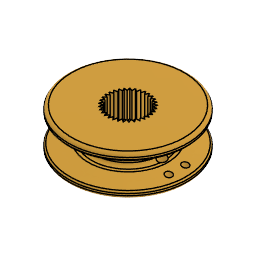
Spool_v3 (Autodesk Fusion 360 design; units mm, degrees)
Autodesk Fusion 360 part; units mm, degrees
sketch "Sketch1" plane through (0, 0, 0) normal (0, 0, 1) x (1, 0, 0)
  line L0 (-0.0246, -2.4999) -> (0.1607, -2.8207)
  line L1 (0.1607, -2.8207) -> (0.3083, -2.4809)
  arc A0 (0.3083, -2.4809) -> (0.449, -2.4594) centre (0, 0) ccw
  line L2 (0.449, -2.4594) -> (0.6916, -2.7393)
  line L3 (0.6916, -2.7393) -> (0.7722, -2.3777)
  arc A1 (0.7722, -2.3777) -> (0.9063, -2.3299) centre (0, 0) ccw
  line L4 (0.9063, -2.3299) -> (1.1975, -2.5589)
  line L5 (1.1975, -2.5589) -> (1.2083, -2.1886)
  arc A2 (1.2083, -2.1886) -> (1.3309, -2.1163) centre (0, 0) ccw
  line L6 (1.3309, -2.1163) -> (1.6601, -2.286)
  line L7 (1.6601, -2.286) -> (1.6006, -1.9204)
  arc A3 (1.6006, -1.9204) -> (1.7073, -1.8262) centre (0, 0) ccw
  line L8 (1.7073, -1.8262) -> (2.0628, -1.9306)
  line L9 (2.0628, -1.9306) -> (1.9351, -1.5828)
  arc A4 (1.9351, -1.5828) -> (2.0221, -1.4701) centre (0, 0) ccw
  line L10 (2.0221, -1.4701) -> (2.3909, -1.5053)
  line L11 (2.3909, -1.5053) -> (2.1997, -1.188)
  arc A5 (2.1997, -1.188) -> (2.2638, -1.0608) centre (0, 0) ccw
  line L12 (2.2638, -1.0608) -> (2.6325, -1.0256)
  line L13 (2.6325, -1.0256) -> (2.3848, -0.7502)
  arc A6 (2.3848, -0.7502) -> (2.4236, -0.6133) centre (0, 0) ccw
  line L14 (2.4236, -0.6133) -> (2.7791, -0.5089)
  line L15 (2.7791, -0.5089) -> (2.4837, -0.2853)
  arc A7 (2.4837, -0.2853) -> (2.4959, -0.1435) centre (0, 0) ccw
  line L16 (2.4959, -0.1435) -> (2.8251, 0.0263)
  line L17 (2.8251, 0.0263) -> (2.4928, 0.1899)
  arc A8 (2.4928, 0.1899) -> (2.4779, 0.3314) centre (0, 0) ccw
  line L18 (2.4779, 0.3314) -> (2.7691, 0.5605)
  line L19 (2.7691, 0.5605) -> (2.4118, 0.6582)
  arc A9 (2.4118, 0.6582) -> (2.3704, 0.7944) centre (0, 0) ccw
  line L20 (2.3704, 0.7944) -> (2.613, 1.0744)
  line L21 (2.613, 1.0744) -> (2.2436, 1.1028)
  arc A10 (2.2436, 1.1028) -> (2.1772, 1.2287) centre (0, 0) ccw
  line L22 (2.1772, 1.2287) -> (2.3625, 1.5495)
  line L23 (2.3625, 1.5495) -> (1.9944, 1.5074)
  arc A11 (1.9944, 1.5074) -> (1.9054, 1.6185) centre (0, 0) ccw
  line L24 (1.9054, 1.6185) -> (2.0265, 1.9686)
  line L25 (2.0265, 1.9686) -> (1.6731, 1.8576)
  arc A12 (1.6731, 1.8576) -> (1.5646, 1.9498) centre (0, 0) ccw
  line L26 (1.5646, 1.9498) -> (1.6173, 2.3165)
  line L27 (1.6173, 2.3165) -> (1.2913, 2.1407)
  arc A13 (1.2913, 2.1407) -> (1.1674, 2.2107) centre (0, 0) ccw
  line L28 (1.1674, 2.2107) -> (1.1497, 2.5807)
  line L29 (1.1497, 2.5807) -> (0.8628, 2.3464)
  arc A14 (0.8628, 2.3464) -> (0.7279, 2.3917) centre (0, 0) ccw
  line L30 (0.7279, 2.3917) -> (0.6405, 2.7517)
  line L31 (0.6405, 2.7517) -> (0.4032, 2.4673)
  arc A15 (0.4032, 2.4673) -> (0.2621, 2.4862) centre (0, 0) ccw
  line L32 (0.2621, 2.4862) -> (0.1082, 2.8232)
  line L33 (0.1082, 2.8232) -> (-0.0711, 2.499)
  arc A16 (-0.0711, 2.499) -> (-0.2132, 2.4909) centre (0, 0) ccw
  line L34 (-0.2132, 2.4909) -> (-0.4281, 2.7926)
  line L35 (-0.4281, 2.7926) -> (-0.5427, 2.4404)
  arc A17 (-0.5427, 2.4404) -> (-0.6807, 2.4055) centre (0, 0) ccw
  line L36 (-0.6807, 2.4055) -> (-0.9488, 2.6612)
  line L37 (-0.9488, 2.6612) -> (-0.9948, 2.2936)
  arc A18 (-0.9948, 2.2936) -> (-1.1237, 2.2332) centre (0, 0) ccw
  line L38 (-1.1237, 2.2332) -> (-1.4353, 2.4335)
  line L39 (-1.4353, 2.4335) -> (-1.4108, 2.0639)
  arc A19 (-1.4108, 2.0639) -> (-1.526, 1.9802) centre (0, 0) ccw
  line L40 (-1.526, 1.9802) -> (-1.8699, 2.1179)
  line L41 (-1.8699, 2.1179) -> (-1.7759, 1.7596)
  arc A20 (-1.7759, 1.7596) -> (-1.8732, 1.6556) centre (0, 0) ccw
  line L42 (-1.8732, 1.6556) -> (-2.2369, 1.7257)
  line L43 (-2.2369, 1.7257) -> (-2.0768, 1.3917)
  arc A21 (-2.0768, 1.3917) -> (-2.1527, 1.2712) centre (0, 0) ccw
  line L44 (-2.1527, 1.2712) -> (-2.5231, 1.2712)
  line L45 (-2.5231, 1.2712) -> (-2.3027, 0.9735)
  arc A22 (-2.3027, 0.9735) -> (-2.3543, 0.8409) centre (0, 0) ccw
  line L46 (-2.3543, 0.8409) -> (-2.7181, 0.7707)
  line L47 (-2.7181, 0.7707) -> (-2.4453, 0.5201)
  arc A23 (-2.4453, 0.5201) -> (-2.4709, 0.3801) centre (0, 0) ccw
  line L48 (-2.4709, 0.3801) -> (-2.8148, 0.2424)
  line L49 (-2.8148, 0.2424) -> (-2.4995, 0.0479)
  arc A24 (-2.4995, 0.0479) -> (-2.4982, -0.0944) centre (0, 0) ccw
  line L50 (-2.4982, -0.0944) -> (-2.8098, -0.2947)
  line L51 (-2.8098, -0.2947) -> (-2.4634, -0.426)
  arc A25 (-2.4634, -0.426) -> (-2.4352, -0.5655) centre (0, 0) ccw
  line L52 (-2.4352, -0.5655) -> (-2.7033, -0.8211)
  line L53 (-2.7033, -0.8211) -> (-2.3383, -0.8845)
  arc A26 (-2.3383, -0.8845) -> (-2.2842, -1.0161) centre (0, 0) ccw
  line L54 (-2.2842, -1.0161) -> (-2.499, -1.3179)
  line L55 (-2.499, -1.3179) -> (-2.1287, -1.311)
  arc A27 (-2.1287, -1.311) -> (-2.0506, -1.4301) centre (0, 0) ccw
  line L56 (-2.0506, -1.4301) -> (-2.2045, -1.767)
  line L57 (-2.2045, -1.767) -> (-1.8421, -1.6902)
  arc A28 (-1.8421, -1.6902) -> (-1.7429, -1.7923) centre (0, 0) ccw
  line L58 (-1.7429, -1.7923) -> (-1.8302, -2.1523)
  line L59 (-1.8302, -2.1523) -> (-1.4889, -2.0083)
  arc A29 (-1.4889, -2.0083) -> (-1.3722, -2.0897) centre (0, 0) ccw
  line L60 (-1.3722, -2.0897) -> (-1.3898, -2.4598)
  line L61 (-1.3898, -2.4598) -> (-1.0819, -2.2538)
  arc A30 (-1.0819, -2.2538) -> (-0.9519, -2.3117) centre (0, 0) ccw
  line L62 (-0.9519, -2.3117) -> (-0.8992, -2.6783)
  line L63 (-0.8992, -2.6783) -> (-0.6359, -2.4178)
  arc A31 (-0.6359, -2.4178) -> (-0.4972, -2.4501) centre (0, 0) ccw
  line L64 (-0.4972, -2.4501) -> (-0.3761, -2.8001)
  line L65 (-0.3761, -2.8001) -> (-0.1668, -2.4944)
  arc A32 (-0.1668, -2.4944) -> (-0.0246, -2.4999) centre (0, 0) ccw
  circle A33 centre (0, 0) radius 9
  circle A34 centre (0, 0) radius 5
  circle A35 centre (5, 0) radius 0.75
  circle A36 centre (0, 0) radius 1.7
  line L66 (7.4, -1.25) -> (7.4, 1.25)
  circle A37 centre (7.4, -1.25) radius 0.5
  circle A38 centre (7.4, 1.25) radius 0.5
  line L67 (7.4, -1.25) -> (7.4, -1.75)
  line L68 (1.728, 2.0321) -> (1.8082, 2.5898)
  line L69 (1.8082, 2.5898) -> (1.3122, 2.3224)
  line L70 (1.3122, 2.3224) -> (1.2854, 2.8852)
  line L71 (1.2854, 2.8852) -> (0.849, 2.5288)
  line L72 (0.849, 2.5288) -> (0.7161, 3.0763)
  line L73 (0.7161, 3.0763) -> (0.3551, 2.6437)
  line L74 (0.3551, 2.6437) -> (0.1209, 3.1563)
  line L75 (0.1209, 3.1563) -> (-0.1517, 2.6632)
  line L76 (-0.1517, 2.6632) -> (-0.4786, 3.1221)
  line L77 (-0.4786, 3.1221) -> (-0.653, 2.5863)
  line L78 (-0.653, 2.5863) -> (-1.0608, 2.9751)
  line L79 (-1.0608, 2.9751) -> (-1.1306, 2.416)
  line L80 (-1.1306, 2.416) -> (-1.6047, 2.7206)
  line L81 (-1.6047, 2.7206) -> (-1.5674, 2.1584)
  line L82 (-1.5674, 2.1584) -> (-2.0905, 2.3678)
  line L83 (-2.0905, 2.3678) -> (-1.9476, 1.8227)
  line L84 (-1.9476, 1.8227) -> (-2.5009, 1.9293)
  line L85 (-2.5009, 1.9293) -> (-2.2573, 1.4212)
  line L86 (-2.2573, 1.4212) -> (-2.8208, 1.4212)
  line L87 (-2.8208, 1.4212) -> (-2.4855, 0.9683)
  line L88 (-2.4855, 0.9683) -> (-3.0388, 0.8617)
  line L89 (-3.0388, 0.8617) -> (-2.6239, 0.4804)
  line L90 (-2.6239, 0.4804) -> (-3.1469, 0.271)
  line L91 (-3.1469, 0.271) -> (-2.6674, -0.0248)
  line L92 (-2.6674, -0.0248) -> (-3.1414, -0.3295)
  line L93 (-3.1414, -0.3295) -> (-2.6145, -0.5292)
  line L94 (-2.6145, -0.5292) -> (-3.0222, -0.918)
  line L95 (-3.0222, -0.918) -> (-2.4671, -1.0144)
  line L96 (-2.4671, -1.0144) -> (-2.7939, -1.4734)
  line L97 (-2.7939, -1.4734) -> (-2.2305, -1.463)
  line L98 (-2.2305, -1.463) -> (-2.4646, -1.9755)
  line L99 (-2.4646, -1.9755) -> (-1.9133, -1.8586)
  line L100 (-1.9133, -1.8586) -> (-2.0462, -2.4062)
  line L101 (-2.0462, -2.4062) -> (-1.527, -2.1872)
  line L102 (-1.527, -2.1872) -> (-1.5538, -2.75)
  line L103 (-1.5538, -2.75) -> (-1.0855, -2.4366)
  line L104 (-1.0855, -2.4366) -> (-1.0053, -2.9943)
  line L105 (-1.0053, -2.9943) -> (-0.6047, -2.598)
  line L106 (-0.6047, -2.598) -> (-0.4204, -3.1305)
  line L107 (-0.4204, -3.1305) -> (-0.1021, -2.6655)
  line L108 (-0.1021, -2.6655) -> (0.1796, -3.1535)
  line L109 (0.1796, -3.1535) -> (0.4042, -2.6367)
  line L110 (0.4042, -2.6367) -> (0.7732, -3.0625)
  line L111 (0.7732, -3.0625) -> (0.8958, -2.5125)
  line L112 (0.8958, -2.5125) -> (1.3388, -2.8608)
  line L113 (1.3388, -2.8608) -> (1.3552, -2.2976)
  line L114 (1.3552, -2.2976) -> (1.856, -2.5558)
  line L115 (1.856, -2.5558) -> (1.7655, -1.9996)
  line L116 (1.7655, -1.9996) -> (2.3061, -2.1583)
  line L117 (2.3061, -2.1583) -> (2.112, -1.6294)
  line L118 (2.112, -1.6294) -> (2.6729, -1.6829)
  line L119 (2.6729, -1.6829) -> (2.3822, -1.2002)
  line L120 (2.3822, -1.2002) -> (2.9431, -1.1466)
  line L121 (2.9431, -1.1466) -> (2.5663, -0.7277)
  line L122 (2.5663, -0.7277) -> (3.1069, -0.5689)
  line L123 (3.1069, -0.5689) -> (2.6576, -0.2289)
  line L124 (2.6576, -0.2289) -> (3.1585, 0.0294)
  line L125 (3.1585, 0.0294) -> (2.6529, 0.2782)
  line L126 (2.6529, 0.2782) -> (3.0958, 0.6266)
  line L127 (3.0958, 0.6266) -> (2.5523, 0.7753)
  line L128 (2.5523, 0.7753) -> (2.9213, 1.2011)
  line L129 (2.9213, 1.2011) -> (2.3595, 1.2443)
  line L130 (2.3595, 1.2443) -> (2.6412, 1.7323)
  line L131 (2.6412, 1.7323) -> (2.0814, 1.6684)
  line L132 (2.0814, 1.6684) -> (2.2656, 2.2008)
  line L133 (2.2656, 2.2008) -> (1.728, 2.0321)
  point P0 (7.4, 0)
  dimension "d1" = 0.15
  dimension "d2" = 18
  dimension "d5" = 10
  dimension "d10" = 1.5
  dimension "d19" = 3.4
  dimension "d24" = 2.5
  dimension "d25" = 1
  dimension "d26" = 1
  constraint concentric A0 A33
  constraint concentric A0 A34
  constraint coincident A34 A35.centre
  constraint concentric A33 A36
  constraint midpoint L66 P0
  constraint vertical L66
  constraint coincident L66.start A37.centre
  constraint coincident L66.end A38.centre
  constraint coincident A37 L67.end
  constraint parallel L66 L67
  measures "d2" diameter of A33
  measures "d5" diameter of A34
  measures "d10" diameter of A35
  measures "d19" diameter of A36
  measures "d24" distance of L66.start L66.end
  measures "d25" diameter of A37
  measures "d26" diameter of A38
extrude "Extrude1" add sketch "Sketch1" along normal blind 6 contours A33 | A34 A35 | A34 A35 | A34 A35 | L66 A37 L67 | L66 A37 L67 | A38
extrude "Extrude2" cut sketch "Sketch1" along normal blind 3 from surface at 1.5 contours A33 | A34 A35 | L66 A37 L67 | L66 A37 L67 | A38 picked at (5.2368, 0.1571)
extrude "Extrude3" cut sketch "Sketch1" along normal blind 4.5 contours L0 L1 A0 L2 L3 A1 L4 L5 A2 L6 L7 A3 L8 L9 A4 L10 L11 A5 L12 L13 A6 L14 L15 A7 L16 L17 A8 L18 L19 A9 L20 L21 A10 L22 L23 A11 L24 L25 A12 L26 L27 A13 L28 L29 A14 L30 L31 A15 L32 L33 A16 L34 L35 A17 L36 L37 A18 L38 L39 A19 L40 L41 A20 L42 L43 A21 L44 L45 A22 L46 L47 A23 L48 L49 A24 L50 L51 A25 L52 L53 A26 L54 L55 A27 L56 L57 A28 L58 L59 A29 L60 L61 A30 L62 L63 A31 L64 L65 A32 | A34 A35 | A34 A35 | A36 | L66 A37 L67 | L66 A37 L67 | A38 | L68 L69 L70 L71 L72 L73 L74 L75 L76 L77 L78 L79 L80 L81 L82 L83 L84 L85 L86 L87 L88 L89 L90 L91 L92 L93 L94 L95 L96 L97 L98 L99 L100 L101 L102 L103 L104 L105 L106 L107 L108 L109 L110 L111 L112 L113 L114 L115 L116 L117 L118 L119 L120 L121 L122 L123 L124 L125 L126 L127 L128 L129 L130 L131 L132 L133 picked at (4.759, 0.1571) picked at (5.2368, 0.1571)
fillet "Fillet2" radius 0.5 2 edges at (-8.3909, -3.2545, 0) (-8.3909, -3.2545, 6)
chamfer "Chamfer1" distance 0.5 distance2 3 2 edges at (-8.3909, 3.2545, 1.5) (-8.3909, -3.2545, 4.5) measured on face at (8.9553, -0.8961, 0.8333) measured on face at (8.9553, -0.8961, 4.8333) tangent chain off
fillet "Fillet4" radius 0.5 2 edges at (-5, 0, 1.5) (-5, 0, 4.5)
extrude "Extrude4" add sketch "Sketch1" along normal blind 2 contours L0 L1 A0 L2 L3 A1 L4 L5 A2 L6 L7 A3 L8 L9 A4 L10 L11 A5 L12 L13 A6 L14 L15 A7 L16 L17 A8 L18 L19 A9 L20 L21 A10 L22 L23 A11 L24 L25 A12 L26 L27 A13 L28 L29 A14 L30 L31 A15 L32 L33 A16 L34 L35 A17 L36 L37 A18 L38 L39 A19 L40 L41 A20 L42 L43 A21 L44 L45 A22 L46 L47 A23 L48 L49 A24 L50 L51 A25 L52 L53 A26 L54 L55 A27 L56 L57 A28 L58 L59 A29 L60 L61 A30 L62 L63 A31 L64 L65 A32 | L68 L69 L70 L71 L72 L73 L74 L75 L76 L77 L78 L79 L80 L81 L82 L83 L84 L85 L86 L87 L88 L89 L90 L91 L92 L93 L94 L95 L96 L97 L98 L99 L100 L101 L102 L103 L104 L105 L106 L107 L108 L109 L110 L111 L112 L113 L114 L115 L116 L117 L118 L119 L120 L121 L122 L123 L124 L125 L126 L127 L128 L129 L130 L131 L132 L133
fillet "Fillet3" radius 0.5 1 edges at (-1.585, 0.6147, 2)
fillet "Fillet5" radius 0.25 2 edges at (-8.3909, -3.2545, 1) (-8.3909, 3.2545, 5)
